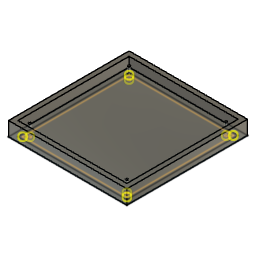
Case_PCB (Autodesk Fusion 360 design; units mm, degrees)
Autodesk Fusion 360 part; units mm, degrees
ref_plane "Plano de trabalho1" through (22.215, 26.505, -5.0525) normal (0, 0, -1) x (-1, 0, 0)
ref_plane "Plano de trabalho2" through (22.215, 26.505, -5.0525) normal (0, 0, -1) x (-1, 0, 0)
sketch "Esboço2" plane through (22.215, 26.505, -5.0525) normal (0, 0, -1) x (1, 0, 0)
  line L0 (22.215, -22.695) -> (22.215, 22.695)
  line L1 (-22.215, -22.695) -> (22.215, -22.695)
  line L2 (-22.215, 22.695) -> (-22.215, -22.695)
  line L3 (22.215, 22.695) -> (-22.215, 22.695)
  circle A0 centre (-20.699, 21.179) radius 0.5
  circle A1 centre (-20.699, -21.179) radius 0.5
  circle A2 centre (20.699, -21.179) radius 0.5
  circle A3 centre (20.699, 21.179) radius 0.5
  line L4 (-25.215, 25.695) -> (-25.215, -25.695)
  line L5 (-25.215, -25.695) -> (25.215, -25.695)
  line L6 (25.215, -25.695) -> (25.215, 25.695)
  line L7 (25.215, 25.695) -> (-25.215, 25.695)
  line L8 (-23.215, 23.695) -> (-23.215, -23.695)
  line L9 (-23.215, -23.695) -> (23.215, -23.695)
  line L10 (23.215, -23.695) -> (23.215, 23.695)
  line L11 (23.215, 23.695) -> (-23.215, 23.695)
  dimension "d19" = 3
  dimension "d20" = 1
extrude "Extrusão8" add sketch "Esboço2" against normal blind 5 contours A3 makes body 1
extrude "Extrusão9" add sketch "Esboço2" against normal blind 5 separate body contours A2 makes body 2
extrude "Extrusão10" add sketch "Esboço2" against normal blind 5 separate body contours A1 makes body 3
extrude "Extrusão11" add sketch "Esboço2" against normal blind 5 separate body contours A0 makes body 4
extrude "Extrusão12" add sketch "Esboço2" against normal blind 5 separate body contours L4 L5 L6 L7 makes body 5
extrude "Extrusão13" add sketch "Esboço2" against normal blind 2 contours L0 L1 L2 L3 | L8 L9 L10 L11 bodies 1 2 3 4 5
extrude "Extrusão14" add 1 faces at (-2.3333, 34.4033, -0.0525) along direction (0, 0, 1) blind 0.5 on bodies 1 bodies 1
extrude "Extrusão15" add 1 faces at (-2.3333, 34.4033, 0.4475) along direction (0, 0, 1) blind 0.5 on bodies 1 bodies 1
